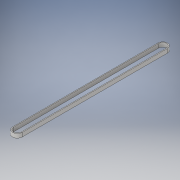
# Autodesk Inventor part: X_Zahnriemen
Saved by Autodesk Inventor 2019 (Build 230136000, 136)
## iProperties
Created: 2018-08-19
Part Number: X_Zahnriemen
Material: Generic
Document SubType Name: Modeling
Designer: Julia
Density: 1 g/cm^3
Appearance: Default
Author: Julia
Autodesk Inventor part; units mm, degrees
ref_plane "YZ Plane" through (0, 0, 0) normal (1, 0, 0) x (0, 1, 0)
ref_plane "XZ Plane" through (0, 0, 0) normal (0, 1, 0) x (-1, 0, 0)
ref_plane "XY Plane" through (0, 0, 0) normal (0, 0, 1) x (1, 0, 0)
sketch "Sketch1" plane through (0, 0, 0) normal (0, 1, 0) x (-1, 0, 0)
  line L0 (0, 288) -> (0, -288) construction
  line L1 (15, 273) -> (15, -273)
  line L2 (-15, -273) -> (-15, 273)
  arc A0 (15, 273) -> (-15, 273) centre (0, 273) ccw
  arc A1 (-15, -273) -> (15, -273) centre (0, -273) ccw
  line L3 (18, -273) -> (18, 273)
  arc A2 (18, 273) -> (-18, 273) centre (0, 273) ccw
  line L4 (-18, 273) -> (-18, -273)
  arc A3 (-18, -273) -> (18, -273) centre (0, -273) ccw
  point P0 (0, 0)
  point P1 (0, 0)
  dimension "d0" = 15
  dimension "d1" = 546
  dimension "d2" = 3
  constraints: 12 end point, 10 point on circle, 4 centre point, 4 tangent, 2 parallel, 2 point on line, 1 coincident, 1 midpoint, 1 vertical, 3 other
  measures "d0" radius of A1
  measures "d1" distance of A0.centre A1.centre
  measures "d2" distance between parallel lines of L1 L3
extrude "Extrusion1" add sketch "Sketch1" along normal blind 15
body "Solid1"
